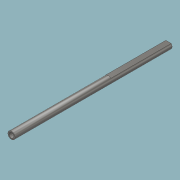
# Autodesk Inventor part: 6mm x 160mm D Shaft
Saved by Autodesk Inventor 2017 SP1 (Build 210196100, 196)
## iProperties
Created: 2018-04-13
Part Number: 6mm x 160mm D Shaft
Material: Stainless Steel
Document SubType Name: Modeling
Designer: Zach
Density: 8 g/cm^3
Appearance: Semi-Polished
Author: Zach
Autodesk Inventor part; units mm, degrees
ref_plane "YZ Plane" through (0, 0, 0) normal (1, 0, 0) x (0, 1, 0)
ref_plane "XZ Plane" through (0, 0, 0) normal (0, 1, 0) x (-1, 0, 0)
ref_plane "XY Plane" through (0, 0, 0) normal (0, 0, 1) x (1, 0, 0)
sketch "Sketch1" plane through (0, 0, 0) normal (0, 0, 1) x (1, 0, 0)
  circle A0 centre (0, 0) radius 3
  line L0 (-2.2361, 2) -> (2.2361, 2)
  arc A1 (-2.2361, 2) -> (2.2361, 2) centre (0, 0) ccw
  dimension "d0" = 6
  dimension "d1" = 2
  constraints: 4 point on circle, 2 centre point, 2 end point, 1 coincident, 1 concentric, 1 horizontal
  measures "d0" diameter of A0
  measures "d1" distance from line of L0 point (0, 0)
extrude "Extrusion1" add sketch "Sketch1" along normal blind 130
sketch "Sketch3" plane through (0, 0, 130) normal (0, 0, 1) x (1, 0, 0)
  circle A0 centre (0, 0) radius 2
  dimension "d22" = 4
  constraints: 1 centre point, 1 coincident
  measures "d22" diameter of A0
extrude "Extrusion3" cut sketch "Sketch3" against normal blind 12.7
sketch "Sketch4" plane through (0, 0, 0) normal (0, 0, -1) x (-1, 0, 0)
  circle A0 centre (0, 0) radius 3 projected
  line L0 (-2.2361, 2) -> (2.2361, 2)
  arc A1 (-2.2361, 2) -> (2.2361, 2) centre (0, 0) ccw
  dimension "d25" = 2
  constraints: 4 point on circle, 2 concentric, 2 end point, 1 centre point, 1 horizontal
  measures "d25" distance from line of point (0, 0) L0
extrude "Extrusion4" cut sketch "Sketch4" against normal blind 50 contours L0 A0 picked at (-0.5653, 2.1582)
body "Solid1"
